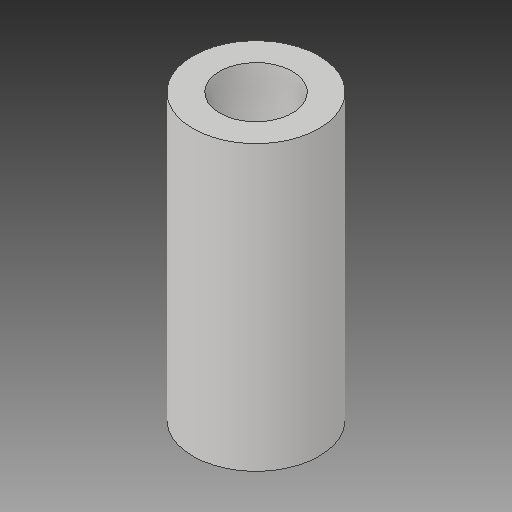
# Autodesk Inventor part: moyeu
Saved by Autodesk Inventor 2019 (Build 230136000, 136)
## iProperties
Created: 2018-03-27
Part Number: moyeu
Material: Générique
Document SubType Name: Modeling
Designer: franc
Density: 1 g/cm^3
Appearance: Par défaut
Author: franc
Autodesk Inventor part; units mm, degrees
ref_plane "YZ Plane" through (0, 0, 0) normal (1, 0, 0) x (0, 1, 0)
ref_plane "XZ Plane" through (0, 0, 0) normal (0, 1, 0) x (-1, 0, 0)
ref_plane "XY Plane" through (0, 0, 0) normal (0, 0, 1) x (1, 0, 0)
sketch "Sketch1" plane through (0, 0, 0) normal (0, 1, 0) x (-1, 0, 0)
  circle A0 centre (0, 0) radius 2
  circle A1 centre (0, 0) radius 1.15
  dimension "d0" = 4
  dimension "d1" = 2.3
  constraints: 2 centre point, 2 coincident
  measures "d0" diameter of A0
  measures "d1" diameter of A1
extrude "Extrusion1" add sketch "Sketch1" along normal blind 9
sketch "Sketch4" plane through (0, 0, 0) normal (1, 0, 0) x (0, 1, 0)
  circle A0 centre (4.5, 0) radius 1
  line L0 (0, 2) -> (0, -2) projected
  point P0 (0, 0)
  dimension "d4" = 2
  dimension "d5" = 4.5
  constraints: 1 centre point
  measures "d4" diameter of A0
  measures "d5" distance from line of L0 A0.centre
extrude "Extrusion2" cut sketch "Sketch4" against normal blind 9
body "Solid1"
